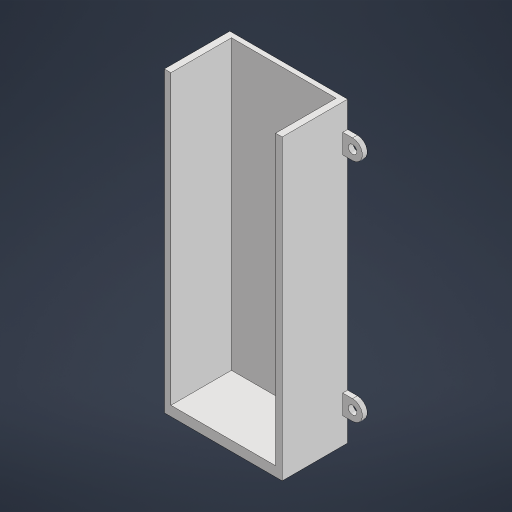
# Autodesk Inventor part: BatteryCase
Saved by Autodesk Inventor 2024.2 (Build 282272000, 272)
## iProperties
Created: 2023-12-22
Part Number: BatteryCase
Material: 一般
Document SubType Name: Modeling
Designer: Hanaoka
Density: 1 g/cm^3
Appearance: 既定
Author: Hanaoka
Autodesk Inventor part; units mm, degrees
ref_plane "YZ Plane" through (0, 0, 0) normal (1, 0, 0) x (0, 1, 0)
ref_plane "XZ Plane" through (0, 0, 0) normal (0, 1, 0) x (-1, 0, 0)
ref_plane "XY Plane" through (0, 0, 0) normal (0, 0, 1) x (1, 0, 0)
sketch "スケッチ1" plane through (0, 0, 0) normal (0, 0, 1) x (1, 0, 0)
  line L0 (18, -45.5) -> (-18, -45.5)
  line L1 (-18, -45.5) -> (-18, 45.5)
  line L2 (-18, 45.5) -> (18, 45.5)
  line L3 (18, 45.5) -> (18, -45.5)
  line L4 (18, -45.5) -> (-18, 45.5) construction
  line L5 (-18, -45.5) -> (18, 45.5) construction
  line L6 (16, 45.5) -> (16, -42.5)
  line L7 (16, -42.5) -> (-16, -42.5)
  line L8 (-16, -42.5) -> (-16, 45.5)
  line L9 (0, -63.7) -> (0, 63.7) projected
  circle A0 centre (-21, -34.5) radius 1.3
  circle A1 centre (-21, 34.5) radius 1.3
  arc A2 (-21, -31.5) -> (-21, -37.5) centre (-21, -34.5) ccw
  line L10 (-21, -37.5) -> (-18, -37.5)
  line L11 (-21, -31.5) -> (-18, -31.5)
  arc A3 (-21, 37.5) -> (-21, 31.5) centre (-21, 34.5) ccw
  line L12 (-21, 31.5) -> (-18, 31.5)
  line L13 (-21, 37.5) -> (-18, 37.5)
  circle A4 centre (21, -34.5) radius 1.3
  circle A5 centre (21, 34.5) radius 1.3
  arc A6 (21, -37.5) -> (21, -31.5) centre (21, -34.5) ccw
  line L14 (21, -37.5) -> (18, -37.5)
  line L15 (21, -31.5) -> (18, -31.5)
  arc A7 (21, 31.5) -> (21, 37.5) centre (21, 34.5) ccw
  line L16 (21, 31.5) -> (18, 31.5)
  line L17 (21, 37.5) -> (18, 37.5)
  point P0 (0, 0)
  dimension "d0" = 36
  dimension "d1" = 3
  dimension "d2" = 2
  dimension "d3" = 88
  dimension "d8" = 2.6
  dimension "d9" = 3
  dimension "d10" = 3
  dimension "d13" = 31.5
  dimension "d14" = 31.5
  constraints: 34 end point, 12 symmetric about line, 10 point on circle, 8 centre point, 6 parallel, 6 point on line, 4 coincident, 4 perpendicular, 4 tangent, 2 equal radius, 2 midpoint, 1 horizontal, 1 vertical, 5 other
  measures "d0" distance of L1.end L2.end
  measures "d1" distance between parallel lines of L7 L0
  measures "d2" distance between parallel lines of L3 L6
  measures "d3" distance of L7.end L8.end
  measures "d8" diameter of A0
  measures "d9" radius of A2
  measures "d10" distance of L11.start L11.end
  measures "d13" distance from line of point (0, 0) L16
  measures "d14" distance from line of point (0, 0) L15
extrude "押し出し1" add sketch "スケッチ1" along normal blind 1.5
extrude "押し出し2" add sketch "スケッチ1" along normal blind 20 contours L0 L9 L7 L6 L2 L3 | L0 L1 L2 L8 L7 L9
equation "\"d14\" = d13"
